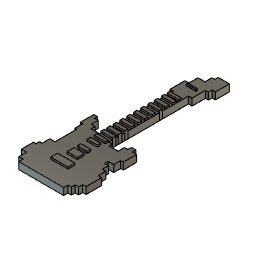
bass_guitar (Autodesk Fusion 360 design; units mm, degrees)
Autodesk Fusion 360 part; units mm, degrees
note: some values were not read from the file. Chosen so that the rebuilt part matches the saved one: which bodies a step acts on; that a step has no effect.
sketch "Sketch1" plane through (0, 0, 0) normal (0, 0, 1) x (1, 0, 0)
sketch "Sketch2" plane through (0, 0, 0) normal (0, 0, 1) x (1, 0, 0)
  line L0 (10.4782, 44.9008) -> (10.4782, 53)
  line L1 (10.4782, 53) -> (4, 53)
  line L2 (4, 53) -> (4, 51)
  line L3 (4, 51) -> (2.3702, 51)
  line L4 (2.3702, 51) -> (2.3702, 46.965)
  line L5 (2.3702, 46.965) -> (-1.6794, 46.965)
  line L6 (-1.6794, 46.965) -> (-1.6794, 45)
  line L7 (-1.6794, 45) -> (-1.6794, 41.6836)
  line L8 (-1.6794, 41.6836) -> (-4, 41.6836)
  line L9 (-4, 41.6836) -> (-4, 33.3866)
  line L10 (-4, 33.3866) -> (-4, 33)
  line L11 (-4, 33) -> (-2, 33)
  line L12 (-2, 33) -> (-2, -9.5731)
  line L13 (-2, -9.5731) -> (-7, -9.5731)
  line L14 (-7, -9.5731) -> (-7, -8)
  line L15 (-7, -8) -> (-7, -7.3)
  line L16 (-7, -7.3) -> (-9.2, -7.3)
  line L17 (-9.2, -7.3) -> (-9.2, -3.2808)
  line L18 (-9.2, -3.2808) -> (-11.2691, -3.2808)
  line L19 (-11.2691, -3.2808) -> (-11.2691, -1.6178)
  line L20 (-11.2691, -1.6178) -> (-13.4093, -1.6178)
  line L21 (-13.4093, -1.6178) -> (-13.4093, -9.3893)
  line L22 (-13.4093, -9.3893) -> (-12, -9.3893)
  line L23 (-12, -9.3893) -> (-12, -14)
  line L24 (-12, -14) -> (-11, -14)
  line L25 (-11, -14) -> (-11, -26.5316)
  line L26 (-11, -26.5316) -> (-12, -26.5316)
  line L27 (-12, -26.5316) -> (-14, -26.5316)
  line L28 (-14, -26.5316) -> (-14, -31)
  line L29 (-14, -31) -> (-15.5274, -31)
  line L30 (-15.5274, -31) -> (-15.5274, -33)
  line L31 (-15.5274, -33) -> (-17, -33)
  line L32 (-17, -33) -> (-17, -40)
  line L33 (-17, -40) -> (-15.5, -40)
  line L34 (-15.5, -40) -> (-14, -40)
  line L35 (-14, -40) -> (-14, -44.5236)
  line L36 (-14, -44.5236) -> (-11.5, -44.5236)
  line L37 (-11.5, -44.5236) -> (-11.5, -47)
  line L38 (-11.5, -47) -> (14.5, -47)
  line L39 (14.5, -47) -> (14.5, -44.5236)
  line L40 (14.5, -44.5236) -> (16.5, -44.5236)
  line L41 (16.5, -44.5236) -> (16.5, -42.4037)
  line L42 (16.5, -42.4037) -> (18.5, -42.4037)
  line L43 (18.5, -42.4037) -> (18.5, -40)
  line L44 (18.5, -40) -> (20.5, -40)
  line L45 (20.5, -40) -> (20.5, -31)
  line L46 (20.5, -31) -> (18.5, -31)
  line L47 (18.5, -31) -> (18.5, -26.5316)
  line L48 (18.5, -26.5316) -> (16.5084, -26.5316)
  line L49 (16.5084, -26.5316) -> (16.5084, -23)
  line L50 (16.5084, -23) -> (14.3308, -23)
  line L51 (14.3308, -23) -> (14.3308, -21)
  line L52 (14.3308, -21) -> (17.5042, -21)
  line L53 (17.5042, -21) -> (17.5042, -17)
  line L54 (17.5042, -17) -> (19, -17)
  line L55 (19, -17) -> (19, -9.2777)
  line L56 (19, -9.2777) -> (16.5, -9.2777)
  line L57 (16.5, -9.2777) -> (16.5, -7.1854)
  line L58 (16.5, -7.1854) -> (14, -7.1854)
  line L59 (14, -7.1854) -> (14, -9.2777)
  line L60 (14, -9.2777) -> (12, -9.2777)
  line L61 (12, -9.2777) -> (12, -13)
  line L62 (12, -13) -> (6.8098, -13)
  line L63 (6.8098, -13) -> (6.8098, -11.1389)
  line L64 (6.8098, -11.1389) -> (4.734, -11.1389)
  line L65 (4.734, -11.1389) -> (4.734, 35)
  line L66 (4.734, 35) -> (6.8098, 35)
  line L67 (6.8098, 35) -> (6.8098, 42.7445)
  line L68 (6.8098, 42.7445) -> (8.5345, 42.7445)
  line L69 (8.5345, 42.7445) -> (8.5345, 44.9033)
  line L70 (8.5345, 44.9033) -> (10.4782, 44.9008)
  line L71 (10.4782, 44.9008) -> (8.5345, 44.9033)
  line L72 (8.5345, 44.9033) -> (8.5345, 44.8225)
  line L73 (8.5345, 44.9033) -> (8.5345, 44.6395)
  line L74 (8.5345, 44.9033) -> (8.5345, 44)
  constraint vertical L0
  constraint perpendicular L0 L1
  constraint perpendicular L1 L2
  constraint perpendicular L2 L3
  constraint perpendicular L3 L4
  constraint perpendicular L5 L6
  constraint perpendicular L5 L7
  constraint perpendicular L7 L8
  constraint perpendicular L8 L9
  constraint horizontal L11
  constraint perpendicular L11 L12
  constraint perpendicular L12 L13
  constraint perpendicular L13 L14
  constraint perpendicular L13 L15
  constraint perpendicular L15 L16
  constraint perpendicular L16 L17
  constraint perpendicular L17 L18
  constraint perpendicular L16 L19
  constraint perpendicular L19 L20
  constraint perpendicular L16 L21
  constraint perpendicular L22 L23
  constraint perpendicular L23 L24
  constraint perpendicular L24 L25
  constraint perpendicular L25 L26
  constraint perpendicular L25 L27
  constraint perpendicular L27 L28
  constraint perpendicular L28 L29
  constraint perpendicular L29 L30
  constraint perpendicular L28 L31
  constraint perpendicular L31 L32
  constraint perpendicular L32 L33
  constraint perpendicular L32 L34
  constraint perpendicular L31 L35
  constraint perpendicular L32 L36
  constraint perpendicular L31 L37
  constraint perpendicular L37 L38
  constraint perpendicular L38 L39
  constraint perpendicular L39 L40
  constraint perpendicular L34 L41
  constraint perpendicular L35 L42
  constraint perpendicular L33 L43
  constraint perpendicular L32 L44
  constraint perpendicular L31 L45
  constraint perpendicular L45 L46
  constraint perpendicular L26 L47
  constraint perpendicular L47 L48
  constraint perpendicular L48 L49
  constraint perpendicular L47 L50
  constraint perpendicular L48 L51
  constraint perpendicular L47 L52
  constraint perpendicular L52 L53
  constraint perpendicular L12 L54
  constraint perpendicular L54 L55
  constraint perpendicular L55 L56
  constraint perpendicular L56 L57
  constraint perpendicular L12 L58
  constraint perpendicular L58 L59
  constraint perpendicular L12 L60
  constraint perpendicular L60 L61
  constraint perpendicular L61 L62
  constraint perpendicular L60 L63
  constraint perpendicular L63 L64
  constraint perpendicular L60 L65
  constraint perpendicular L0 L66
  constraint perpendicular L66 L67
  constraint perpendicular L67 L68
  constraint perpendicular L68 L69
  constraint parallel L70 L71
  constraint coincident L69 L72.end
  constraint coincident L69 L73.end
  constraint coincident L69 L74.end
sketch "Sketch3" plane through (0, 0, 0) normal (0, 0, 1) x (1, 0, 0)
sketch "Sketch4" plane through (0, 0, 0) normal (0, 0, 1) x (1, 0, 0)
  line L0 (-3.5, -32.5) -> (-3.5, -36.5)
  line L1 (-3.5, -36.5) -> (6.5, -36.5)
  line L2 (6.5, -36.5) -> (6.5, -32.5)
  line L3 (6.5, -32.5) -> (-3.5, -32.5)
  line L4 (-1.4946, -24.9067) -> (-1.4946, -29)
  line L5 (-1.4946, -29) -> (4.4098, -29)
  line L6 (4.4098, -29) -> (4.4098, -25)
  line L7 (-1.4946, -24.9067) -> (4.4098, -24.9067)
  line L8 (4.4098, -25) -> (4.4098, -24.9067)
  constraint vertical L0
  constraint perpendicular L0 L1
  constraint perpendicular L1 L2
  constraint perpendicular L0 L3
  constraint perpendicular L3 L4
  constraint perpendicular L4 L5
  constraint perpendicular L5 L6
  constraint perpendicular L6 L7
  constraint perpendicular L7 L8
sketch "Sketch5" plane through (0, 0, 0) normal (0, 0, 1) x (1, 0, 0)
  line L0 (-1.5, -21) -> (-1.5, -23)
  line L1 (-1.5, -23) -> (4.2102, -23)
  line L2 (4.2102, -23) -> (4.2102, -21)
  line L3 (4.2102, -21) -> (-1.5, -21)
  constraint vertical L0
  constraint perpendicular L0 L1
  constraint perpendicular L1 L2
  constraint perpendicular L0 L3
sketch "Sketch6" plane through (0, 0, 0) normal (0, 0, 1) x (1, 0, 0)
  line L0 (-2, -15) -> (-2, -17)
  line L1 (-2, -17) -> (4, -17)
  line L2 (4, -17) -> (4, -15)
  line L3 (4, -15) -> (-2, -15)
  line L4 (-1.9482, -13) -> (4.6272, -13)
  line L5 (4.6272, -13) -> (4.6272, -11.2516)
  line L6 (4.6272, -11.2516) -> (-1.9482, -11.2516)
  line L7 (-1.9482, -11.2516) -> (-1.9482, -13)
  line L8 (-2, -9) -> (4.7353, -9)
  line L9 (4.7353, -9) -> (4.7353, -7)
  line L10 (4.7353, -7) -> (-2, -7)
  line L11 (-2, -7) -> (-2, -9)
  line L12 (-2, -5.6536) -> (4.7619, -5.6536)
  line L13 (4.7619, -5.6536) -> (4.7619, -3.5043)
  line L14 (4.7619, -3.5043) -> (-2, -3.5043)
  line L15 (-2, -3.5043) -> (-2, -5.6536)
  line L16 (-2, -1.8725) -> (4.735, -1.8725)
  line L17 (4.735, -1.8725) -> (4.735, 0)
  line L18 (4.735, 0) -> (-2, 0)
  line L19 (-2, 0) -> (-2, -1.8725)
  line L20 (-2, 1.9829) -> (4.7264, 1.9829)
  line L21 (4.7264, 1.9829) -> (4.7264, 4)
  line L22 (4.7264, 4) -> (-2, 4)
  line L23 (-2, 4) -> (-2, 1.9829)
  line L24 (-2, 6.0107) -> (4.7339, 6.0107)
  line L25 (4.7339, 6.0107) -> (4.7339, 8)
  line L26 (4.7339, 8) -> (-2, 8)
  line L27 (-2, 8) -> (-2, 6.0107)
  line L28 (4.4456, 10.0046) -> (-2, 10.0046)
  line L29 (-2, 10.0046) -> (-2, 12)
  line L30 (-2, 12) -> (4.4456, 12)
  line L31 (4.4456, 12) -> (4.4456, 10.0046)
  line L32 (4.7296, 14.0403) -> (-2, 14.0403)
  line L33 (-2, 14.0403) -> (-2, 16)
  line L34 (-2, 16) -> (4.7296, 16)
  line L35 (4.7296, 16) -> (4.7296, 14.0403)
  line L36 (4.7364, 18.2235) -> (-2, 18.2235)
  line L37 (-2, 18.2235) -> (-2, 20)
  line L38 (-2, 20) -> (4.7364, 20)
  line L39 (4.7364, 20) -> (4.7364, 18.2235)
  line L40 (4.7237, 21.9364) -> (-2, 21.9364)
  line L41 (-2, 21.9364) -> (-2, 24)
  line L42 (-2, 24) -> (4.7237, 24)
  line L43 (4.7237, 24) -> (4.7237, 21.9364)
  line L44 (4.7237, 26.0741) -> (4, 26.0741)
  line L45 (4, 26.0741) -> (-2, 26.0741)
  line L46 (-2, 26.0741) -> (-2, 28)
  line L47 (-2, 28) -> (4.7237, 28)
  line L48 (4.7237, 28) -> (4.7237, 26.0741)
  line L49 (4.7143, 29.3687) -> (-2, 29.3687)
  line L50 (-2, 29.3687) -> (-2, 31)
  line L51 (-2, 31) -> (4.7143, 31)
  line L52 (4.7143, 31) -> (4.7143, 29.3687)
  constraint vertical L0
  constraint perpendicular L0 L1
  constraint perpendicular L1 L2
  constraint perpendicular L0 L3
  constraint perpendicular L0 L4
  constraint perpendicular L4 L5
  constraint perpendicular L0 L6
  constraint perpendicular L4 L7
  constraint perpendicular L7 L8
  constraint perpendicular L8 L9
  constraint perpendicular L9 L10
  constraint perpendicular L8 L11
  constraint perpendicular L11 L12
  constraint perpendicular L10 L13
  constraint perpendicular L13 L14
  constraint perpendicular L14 L15
  constraint perpendicular L15 L16
  constraint perpendicular L16 L17
  constraint perpendicular L15 L18
  constraint perpendicular L16 L19
  constraint perpendicular L19 L20
  constraint perpendicular L18 L21
  constraint perpendicular L19 L22
  constraint perpendicular L20 L23
  constraint perpendicular L23 L24
  constraint perpendicular L24 L25
  constraint perpendicular L25 L26
  constraint perpendicular L26 L27
  constraint perpendicular L25 L28
  constraint perpendicular L26 L29
  constraint perpendicular L29 L30
  constraint perpendicular L28 L31
  constraint perpendicular L31 L32
  constraint perpendicular L30 L33
  constraint perpendicular L33 L34
  constraint perpendicular L32 L35
  constraint perpendicular L35 L36
  constraint perpendicular L36 L37
  constraint perpendicular L37 L38
  constraint perpendicular L36 L39
  constraint perpendicular L39 L40
  constraint perpendicular L40 L41
  constraint perpendicular L41 L42
  constraint perpendicular L40 L43
  constraint perpendicular L43 L44
  constraint perpendicular L43 L45
  constraint perpendicular L45 L46
  constraint perpendicular L46 L47
  constraint perpendicular L44 L48
  constraint perpendicular L48 L49
  constraint perpendicular L44 L50
  constraint perpendicular L48 L51
  constraint perpendicular L49 L52
sketch "Sketch7" plane through (0, 0, 0) normal (0, 0, 1) x (1, 0, 0)
sketch "Sketch8" plane through (0, 0, 0) normal (0, 0, 1) x (1, 0, 0)
sketch "Sketch9" plane through (0, 0, 0) normal (0, 0, 1) x (1, 0, 0)
  line L0 (-0.1955, 39.9817, 10) -> (-0.6401, 39.9817, 10)
  line L1 (-0.6401, 39.9817, 10) -> (-0.6401, -34, 10)
  line L2 (-0.6401, -34, 10) -> (-0.1955, -34, 10)
  line L3 (-0.1955, -34, 10) -> (-0.1955, 39.9817, 10)
sketch "Sketch10" plane through (0, 0, 0) normal (0, 0, 1) x (1, 0, 0)
sketch "Sketch11" plane through (0, 0, 0) normal (0, 0, 1) x (1, 0, 0)
  line L0 (-1, 40.2953) -> (4.6081, 40.2953)
  line L1 (4.6081, 40.2953) -> (4.6081, 39.5)
  line L2 (4.6081, 39.5) -> (-1, 39.5)
  line L3 (-1, 39.5) -> (-1, 40.2953)
  constraint horizontal L0
  constraint vertical L1
  constraint horizontal L2
  constraint vertical L3
sketch "Sketch12" plane through (0, 0, 0) normal (0, 0, 1) x (1, 0, 0)
sketch "Sketch13" plane through (0, 0, 0) normal (0, 0, 1) x (1, 0, 0)
sketch "Sketch14" plane through (0, 0, 0) normal (0, 0, 1) x (1, 0, 0)
sketch "Sketch15" plane through (0, 0, 0) normal (0, 0, 1) x (1, 0, 0)
sketch "Sketch16" plane through (0, 0, 0) normal (0, 0, 1) x (1, 0, 0)
  line L0 (-1.6796, 43) -> (-3.5, 43)
  line L1 (-3.5, 43) -> (-3.5, 45)
  line L2 (-3.5, 45) -> (-1.6796, 45)
  line L3 (-1.6796, 45) -> (-1.6796, 43)
  constraint horizontal L0
  constraint vertical L1
  constraint horizontal L2
  constraint vertical L3
sketch "Sketch17" plane through (0, 0, 0) normal (0, 0, 1) x (1, 0, 0)
  line L0 (2.37, 48.9858) -> (-1.5761, 48.9858)
  line L1 (-1.5761, 48.9858) -> (-1.5761, 46.965)
  line L2 (-1.5761, 46.965) -> (2.37, 46.965)
  line L3 (2.37, 46.965) -> (2.37, 48.9858)
  constraint horizontal L0
  constraint vertical L1
  constraint horizontal L2
  constraint vertical L3
sketch "Sketch18" plane through (0, 0, 0) normal (0, 0, 1) x (1, 0, 0)
  line L0 (-5.5608, 41.3211) -> (-4, 41.3211)
  line L1 (-4, 41.3211) -> (-4, 39)
  line L2 (-4, 39) -> (-5.5608, 39)
  line L3 (-5.5608, 39) -> (-5.5608, 41.3211)
  line L4 (-5.5608, 37.353) -> (-4, 37.353)
  line L5 (-4, 37.353) -> (-4, 35)
  line L6 (-4, 35) -> (-5.5608, 35)
  line L7 (-5.5608, 35) -> (-5.5608, 37.353)
  constraint horizontal L0
  constraint vertical L1
  constraint horizontal L2
  constraint vertical L3
  constraint horizontal L4
  constraint vertical L5
  constraint horizontal L6
  constraint vertical L7
sketch "Sketch19" plane through (0, 0, 0) normal (0, 0, 1) x (1, 0, 0)
extrude "Extrude1" add sketch "Sketch4" sketch "Sketch5" sketch "Sketch6" sketch "Sketch11" along normal blind 5 of sketch 2 of sketch 3 of sketch 4 makes body 1 at (2.4843, 4, 1.6667) makes body 2 at (0.2432, 16, 1.6667) makes body 3 at (0.2381, 31, 1.6667) makes body 4 at (2, -15, 1.6667) makes body 5 at (2.5079, -3.5043, 3.3333) makes body 6 at (2.4909, 18.2235, 1.6667) makes body 7 at (2.49, 0, 1.6667) makes body 8 at (2.4417, -24.9067, 3.3333) makes body 9 at (3.1667, -32.5, 1.6667) makes body 10 at (0.4034, -21, 3.3333) makes body 11 at (2.2971, 10.0046, 1.6667) makes body 12 at (2.4825, 28, 3.3333) makes body 13 at (0.2436, -13, 1.6667) makes body 14 at (2.4902, -7, 1.6667) makes body 15 at (2.4825, 21.9364, 1.6667) makes body 16 at (2.4893, 8, 1.6667) makes body 17 at (0.8694, 40.2953, 1.6667)
extrude "Extrude2" add sketch "Sketch2" along normal blind 4 bodies 1 2 3 4 5 6 7 8 9 10 11 12 13 14 15 16 17
form "Form1" [no effect]
sketch "Sketch20" plane through (0, 0, 0) normal (0, 0, 1) x (1, 0, 0)
  line L0 (0.4203, 39.999) -> (0.4203, -34)
  line L1 (0.4203, -34) -> (1, -34)
  line L2 (1, -34) -> (0.8373, 39.999)
  line L3 (0.8373, 39.999) -> (0.4203, 39.999)
  constraint vertical L0
  constraint perpendicular L0 L1
  constraint perpendicular L0 L3
sketch "Sketch21" plane through (0, 0, 0) normal (0, 0, 1) x (1, 0, 0)
sketch "Sketch22" plane through (0, 0, 0) normal (0, 0, 1) x (1, 0, 0)
  line L0 (1.4175, 40.0514) -> (1.8103, 40.0514)
  line L1 (1.8103, 40.0514) -> (1.8103, -34)
  line L2 (1.8103, -34) -> (1.4175, -34)
  line L3 (1.4175, -34) -> (1.4175, 40.0514)
  constraint horizontal L0
  constraint vertical L1
  constraint horizontal L2
  constraint vertical L3
sketch "Sketch23" plane through (0, 0, 0) normal (0, 0, 1) x (1, 0, 0)
  line L0 (2.172, 40) -> (2.4973, 40)
  line L1 (2.4973, 40) -> (2.4973, -34)
  line L2 (2.4973, -34) -> (2.172, -34)
  line L3 (2.172, -34) -> (2.172, 40)
  constraint horizontal L0
  constraint vertical L1
  constraint horizontal L2
  constraint vertical L3
sketch "Sketch24" plane through (0, 0, 3) normal (0, 0, 1) x (-1, 0, 0)
  line L0 (-0.8373, -39.999) -> (-0.4203, -39.999)
  line L1 (-0.4203, -39.999) -> (-0.4203, 34)
  line L2 (-0.4203, 34) -> (-1, 34)
  line L3 (-1, 34) -> (-0.8373, -39.999)
sketch "Sketch25" plane through (0, 0, 0) normal (0, 0, 1) x (1, 0, 0)
sketch "Sketch26" plane through (0, 0, 0) normal (0, 0, 1) x (1, 0, 0)
sketch "Sketch27" plane through (0, -47, 0) normal (0, -1, 0) x (1, 0, 0)
  line L0 (-11.5, 0) -> (14.5, 0)
  line L1 (14.5, 0) -> (14.5, 4)
  line L2 (14.5, 4) -> (-11.5, 4)
  line L3 (-11.5, 4) -> (-11.5, 0)
component "Component" placed x (1, 0, 0) y (0, 1, 0) z (0, 0, 1) at (0, 0, 0)
